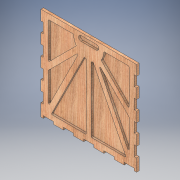
# Autodesk Inventor part: SizingCrateMajorSide
Saved by Autodesk Inventor 2017.3 (Build 213256000, 256)
## iProperties
Created: 2019-04-26
Part Number: SizingCrateMajorSide
Material: Wood (Birch)
Document SubType Name: Modeling
Designer: guberti
Density: 0.55 g/cm^3
Appearance: Birch - Natural Polished
Mass: 895.197 g
Surface Area: 5075.85 cm^2
Volume: 1627.63 cm^3
Author: guberti
Autodesk Inventor part; units mm, degrees
ref_plane "YZ Plane" through (0, 0, 0) normal (1, 0, 0) x (0, 1, 0)
ref_plane "XZ Plane" through (0, 0, 0) normal (0, 1, 0) x (-1, 0, 0)
ref_plane "XY Plane" through (0, 0, 0) normal (0, 0, 1) x (1, 0, 0)
sketch "Sketch1" plane through (0, 0, 0) normal (0, 0, 1) x (1, 0, 0)
  line L0 (0, 0) -> (0, -11.9062)
  line L1 (0, -11.9062) -> (-11.9062, -11.9062)
  line L2 (0, 0) -> (50.8, 0)
  line L3 (50.8, 0) -> (50.8, -11.9062)
  line L4 (50.8, -11.9062) -> (101.6, -11.9062)
  line L5 (101.6, -11.9062) -> (101.6, 0)
  line L6 (101.6, 0) -> (152.4, 0)
  line L7 (152.4, 0) -> (152.4, -11.9062)
  line L8 (152.4, -11.9062) -> (203.2, -11.9062)
  line L9 (203.2, -11.9062) -> (203.2, 0)
  line L10 (-11.9062, -11.9062) -> (-11.9062, 50.8)
  line L11 (-11.9062, 50.8) -> (0, 50.8)
  line L12 (0, 50.8) -> (0, 101.6)
  line L13 (0, 101.6) -> (-11.9062, 101.6)
  line L14 (-11.9062, 101.6) -> (-11.9062, 152.4)
  line L15 (-11.9062, 152.4) -> (0, 152.4)
  line L16 (0, 152.4) -> (0, 203.2)
  line L17 (0, 203.2) -> (-11.9062, 203.2)
  line L18 (-11.9062, 203.2) -> (-11.9062, 254)
  line L19 (-11.9062, 254) -> (0, 254)
  line L20 (0, 254) -> (0, 304.8)
  line L21 (0, 304.8) -> (-11.9062, 304.8)
  line L22 (-11.9062, 304.8) -> (-11.9062, 355.6)
  line L23 (-11.9062, 355.6) -> (0, 355.6)
  line L24 (0, 355.6) -> (0, 406.4)
  line L25 (0, 406.4) -> (-11.9062, 406.4)
  line L26 (-11.9062, 406.4) -> (-11.9062, 457.2)
  line L27 (228.6, 0) -> (228.6, 457.2) construction
  line L28 (457.2, 0) -> (457.2, -11.9062)
  line L29 (457.2, -11.9062) -> (469.1063, -11.9062)
  line L30 (457.2, 0) -> (406.4, 0)
  line L31 (406.4, 0) -> (406.4, -11.9062)
  line L32 (406.4, -11.9062) -> (355.6, -11.9062)
  line L33 (355.6, -11.9062) -> (355.6, 0)
  line L34 (355.6, 0) -> (304.8, 0)
  line L35 (304.8, 0) -> (304.8, -11.9062)
  line L36 (304.8, -11.9062) -> (254, -11.9062)
  line L37 (254, -11.9062) -> (254, 0)
  line L38 (469.1063, -11.9062) -> (469.1063, 50.8)
  line L39 (469.1063, 50.8) -> (457.2, 50.8)
  line L40 (457.2, 50.8) -> (457.2, 101.6)
  line L41 (457.2, 101.6) -> (469.1063, 101.6)
  line L42 (469.1063, 101.6) -> (469.1063, 152.4)
  line L43 (469.1063, 152.4) -> (457.2, 152.4)
  line L44 (457.2, 152.4) -> (457.2, 203.2)
  line L45 (457.2, 203.2) -> (469.1063, 203.2)
  line L46 (469.1063, 203.2) -> (469.1063, 254)
  line L47 (469.1063, 254) -> (457.2, 254)
  line L48 (457.2, 254) -> (457.2, 304.8)
  line L49 (457.2, 304.8) -> (469.1063, 304.8)
  line L50 (469.1063, 304.8) -> (469.1063, 355.6)
  line L51 (469.1063, 355.6) -> (457.2, 355.6)
  line L52 (457.2, 355.6) -> (457.2, 406.4)
  line L53 (457.2, 406.4) -> (469.1063, 406.4)
  line L54 (469.1063, 406.4) -> (469.1063, 457.2)
  line L55 (203.2, 0) -> (254, 0)
  line L56 (-11.9062, 457.2) -> (469.1063, 457.2)
  dimension "thickness" = 11.9062
  dimension "toothwidth" = 50.8
  dimension "d10" = 62.7062
  dimension "d26" = 457.2
  dimension "d27" = 228.6
  constraints: 114 end point, 28 symmetric about line, 24 equal length, 22 point on line, 10 perpendicular, 6 vertical, 2 horizontal, 1 midpoint, 1 parallel
  measures "thickness" distance of L0.start L0.end
  measures "toothwidth" distance of L0.start L2.end
  measures "d10" distance of L1.end L10.end
  measures "d26" distance of L27.start L27.end
  measures "d27" distance between parallel lines of L20 L27
extrude "Extrusion1" add sketch "Sketch1" along normal blind 12.7
sketch "Sketch2" plane through (0, 0, 12.7) normal (0, 0, 1) x (1, 0, 0)
  line L0 (26.1938, 26.1938) -> (431.0062, 26.1938) construction
  line L1 (431.0062, 26.1938) -> (431.0062, 431.0063) construction
  line L2 (431.0062, 431.0063) -> (26.1938, 431.0063) construction
  line L3 (26.1938, 431.0063) -> (26.1938, 26.1938) construction
  line L4 (469.1063, 457.2) -> (-11.9062, 457.2) construction
  line L5 (-11.9062, 355.6) -> (-11.9062, 304.8) construction
  line L6 (152.4, -11.9062) -> (203.2, -11.9062) construction
  line L7 (469.1063, 203.2) -> (469.1063, 254) projected
  line L8 (190.5, 431.0062) -> (266.7, 431.0062) construction
  line L9 (190.5, 418.3062) -> (266.7, 418.3062)
  line L10 (266.7, 443.7063) -> (190.5, 443.7062)
  arc A0 (190.5, 443.7062) -> (190.5, 418.3062) centre (190.5, 431.0062) ccw
  arc A1 (266.7, 418.3062) -> (266.7, 443.7063) centre (266.7, 431.0062) ccw
  line L11 (-11.9062, 457.2) -> (469.1063, 457.2) projected
  line L12 (26.1937, 228.6) -> (228.6, 431.0062) construction
  line L13 (228.6, 431.0062) -> (26.1938, 26.1938) construction
  line L14 (431.0063, 228.6) -> (228.6, 431.0062) construction
  line L15 (431.0062, 26.1938) -> (228.6, 431.0062) construction
  line L16 (228.6, 26.1938) -> (228.6, 431.0062) construction
  line L17 (166.4918, 386.8586) -> (26.1937, 246.5605)
  line L18 (26.1938, 210.6395) -> (168.296, 352.7418)
  line L19 (206.3582, 358.1246) -> (40.3928, 26.1938)
  line L20 (26.1938, 54.5918) -> (173.4216, 349.0475)
  line L21 (241.3, 26.1937) -> (241.3, 355.872)
  line L22 (215.9, 355.872) -> (215.9, 26.1938)
  line L23 (431.0063, 54.5918) -> (283.7784, 349.0475)
  line L24 (250.8418, 358.1246) -> (416.8072, 26.1938)
  line L25 (431.0062, 246.5605) -> (290.7082, 386.8586)
  line L26 (288.904, 352.7418) -> (431.0062, 210.6395)
  line L27 (304.8, 431.0062) -> (431.0062, 431.0063)
  line L28 (431.0062, 431.0063) -> (431.0062, 246.5605)
  line L29 (431.0062, 210.6395) -> (431.0063, 54.5918)
  line L30 (416.8072, 26.1938) -> (241.3, 26.1937)
  line L31 (215.9, 26.1938) -> (40.3928, 26.1938)
  line L32 (26.1938, 54.5918) -> (26.1938, 210.6395)
  line L33 (152.4, 431.0063) -> (26.1938, 431.0063)
  line L34 (26.1938, 431.0063) -> (26.1937, 246.5605)
  arc A2 (173.4216, 349.0475) -> (168.296, 352.7418) centre (170.5591, 350.4788) ccw
  arc A3 (288.904, 352.7418) -> (283.7784, 349.0475) centre (286.6409, 350.4788) ccw
  arc A4 (290.7082, 386.8586) -> (304.8, 431.0062) centre (228.6, 431.0062) ccw
  arc A5 (241.3, 355.872) -> (250.8418, 358.1246) centre (228.6, 431.0062) ccw
  arc A6 (152.4, 431.0063) -> (166.4918, 386.8586) centre (228.6, 431.0062) ccw
  arc A7 (206.3582, 358.1246) -> (215.9, 355.872) centre (228.6, 431.0062) ccw
  point P0 (0, 0)
  dimension "d30" = 26.1938
  dimension "border" = 38.1
  dimension "d33" = 38.1
  dimension "d34" = 38.1
  dimension "d35" = 38.1
  dimension "d36" = 25.4
  dimension "strutrad" = 12.7
  dimension "d38" = 12.7
  dimension "d39" = 12.7
  dimension "d40" = 12.7
  dimension "d41" = 12.7
  dimension "d42" = 12.7
  dimension "d43" = 12.7
  dimension "d44" = 12.7
  dimension "d45" = 12.7
  dimension "d46" = 12.7
  dimension "bitrad" = 3.2004
  dimension "d48" = 3.2004
  dimension "circrad" = 76.2
  dimension "d50" = 76.2
  dimension "d51" = 76.2
  dimension "d52" = 76.2
  constraints: 62 end point, 16 point on circle, 13 point on line, 12 parallel, 8 centre point, 8 tangent, 6 collinear, 5 midpoint, 4 perpendicular, 2 coincident, 1 horizontal, 1 vertical
  measures "d30" distance between parallel lines of L4 L2
  measures "border" distance between parallel lines of L5 L3
  measures "d33" distance between parallel lines of L6 L0
  measures "d34" distance between parallel lines of L7 L1
  measures "d35" distance of point (228.6, 431.006) L8.end
  measures "d36" diameter of A1
  measures "strutrad" distance between parallel lines of L17 L12
  measures "d38" distance between parallel lines of L18 L12
  measures "d39" distance between parallel lines of L20 L13
  measures "d40" distance between parallel lines of L19 L13
  measures "d41" distance between parallel lines of L21 L16
  measures "d42" distance between parallel lines of L22 L16
  measures "d43" distance between parallel lines of L15 L23
  measures "d44" distance between parallel lines of L24 L15
  measures "d45" distance between parallel lines of L25 L14
  measures "d46" distance between parallel lines of L26 L14
  measures "bitrad" radius of A2
  measures "d48" radius of A3
  measures "circrad" radius of A6
  measures "d50" radius of A7
  measures "d51" radius of A5
  measures "d52" radius of A4
extrude "Extrusion2" cut sketch "Sketch2" against normal blind 9.525
fillet "Fillet1" radius 3.2004 20 edges at (206.3582, 358.1246, 7.9375) (215.9, 355.872, 7.9375) (152.4, 431.0063, 7.9375) (26.1938, 431.0063, 7.9375) (26.1937, 246.5605, 7.9375) (26.1938, 210.6395, 7.9375) (26.1938, 54.5918, 7.9375) (40.3928, 26.1938, 7.9375) (215.9, 26.1938, 7.9375) (241.3, 26.1937, 7.9375) (416.8072, 26.1938, 7.9375) (431.0063, 54.5918, 7.9375) (250.8418, 358.1246, 7.9375) (241.3, 355.872, 7.9375) (304.8, 431.0062, 7.9375) (290.7082, 386.8586, 7.9375) (431.0062, 431.0063, 7.9375) (431.0062, 246.5605, 7.9375) (431.0062, 210.6395, 7.9375) (166.4918, 386.8586, 7.9375)
equation "\"d10\" = toothwidth + thickness"
equation "\"d30\" = border - thickness"
equation "\"d33\" = border"
equation "\"d38\" = strutrad"
equation "\"d39\" = strutrad"
equation "\"d40\" = strutrad"
equation "\"d41\" = strutrad"
equation "\"d42\" = strutrad"
equation "\"d43\" = strutrad"
equation "\"d44\" = strutrad"
equation "\"d45\" = strutrad"
equation "\"d46\" = strutrad"
equation "\"d48\" = bitrad"
equation "\"d50\" = circrad"
equation "\"d51\" = circrad"
equation "\"d52\" = circrad"
equation "\"d55\" = bitrad"
body "Solid1"
